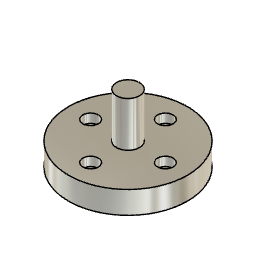
Full Assembly v48 (Autodesk Fusion 360 archive; units mm, degrees)
design "Top Cap For Metal Cylinder"
Autodesk Fusion 360 part; units mm, degrees
cylinder "CylinderPrimitive1" add diameter 50.5 height 28.575 placed x (1, 0, 0) y (0, 1, 0) z (0, 0, 1) at (0, 0, 0)
sketch "Sketch2" plane through (0, 0, 28.575) normal (0, 0, 1) x (-1, 0, 0)
  circle A0 centre (0, 0) radius 25.25
  circle A1 centre (0, 0) radius 4.9
  dimension "d3" = 9.8
  constraint concentric A0 A1
  measures "d3" diameter of A1
extrude "Extrude1" cut sketch "Sketch2" against normal blind 19.05
sketch "Sketch3" plane through (0, 0, 9.525) normal (0, 0, 1) x (-1, 0, 0)
  circle A0 centre (0, 0) radius 4.9
  circle A1 centre (0, 0) radius 25.25
  line L0 (0, 0) -> (0, 15.875)
  line L1 (0, 0) -> (15.875, 0)
  line L2 (0, 0) -> (0, -15.875)
  line L3 (0, 0) -> (-15.875, 0)
  dimension "d6" = 15.875
  dimension "d7" = 15.875
  dimension "d8" = 15.875
  dimension "d9" = 15.875
  constraint coincident A0.centre A1.centre
  constraint vertical L0
  constraint horizontal L1
  constraint vertical L2
  constraint perpendicular L2 L3
  measures "d6" distance of A0.centre L0.end
  measures "d7" distance of A0.centre L1.end
  measures "d8" distance of A0.centre L2.end
  measures "d9" distance of A0.centre L3.end
hole "Hole1" at (-15.875, 0, 9.525) at (0, 15.875, 9.525) at (0, -15.875, 9.525) at (15.875, 0, 9.525) direction (0, 0, -1) diameter 3.9 depth 16.3 tip angle 180 counterbore diameter 6.6 counterbore depth 3.8

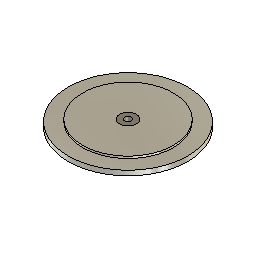
design "Top Rotary Disk"
Autodesk Fusion 360 part; units mm, degrees
sketch "Sketch1" plane through (0, 0, 0) normal (0, 0, 1) x (1, 0, 0)
  circle A0 centre (0, 0) radius 89
  circle A1 centre (0, 0) radius 67.55
  dimension "d1" = 178
  dimension "d2" = 135.1
  constraint coincident A0.centre A1.centre
  measures "d1" diameter of A0
  measures "d2" diameter of A1
extrude "Extrude1" add sketch "Sketch1" along normal blind 8 contours A1 makes body 1
extrude "Extrude2" add sketch "Sketch1" along normal blind 5 bodies 1
sketch "Sketch2" plane through (0, 0, 8) normal (0, 0, 1) x (-1, 0, 0)
  circle A0 centre (0, 0) radius 67.55
  circle A1 centre (0, 0) radius 12.5
  circle A2 centre (0, 0) radius 4.9
  dimension "d7" = 25
  dimension "d19" = 9.8
  constraint coincident A0.centre A1.centre
  measures "d7" diameter of A1
  measures "d19" diameter of A2
extrude "Extrude3" cut sketch "Sketch2" against normal blind 10 contours A1 | A2 bodies 1
sketch "Sketch3" plane through (0, 0, 0) normal (0, 0, 1) x (1, 0, 0)
  circle A0 centre (0, 0) radius 4.9
  circle A1 centre (0, 0) radius 12.5
  dimension "d10" = 9.8
  constraint coincident A0.centre A1.centre
  measures "d10" diameter of A0
extrude "Extrude5" add sketch "Sketch1" against normal blind 2.1882 contours A0 | A1 bodies 1
sketch "Sketch4" plane through (0, 0, -2.1882) normal (0, 0, -1) x (1, 0, 0)
  circle A0 centre (0, 0) radius 89
  circle A1 centre (0, 0) radius 19.05
  circle A2 centre (0, 0) radius 5.08
  dimension "d15" = 38.1
  dimension "d16" = 10.16
  constraint coincident A0.centre A1.centre
  measures "d15" diameter of A1
  measures "d16" diameter of A2
extrude "Extrude6" add sketch "Sketch4" along normal blind 12.7 contours A1 bodies 1
sketch "Sketch5" plane through (0, 0, 8) normal (0, 0, 1) x (-1, 0, 0)
  circle A0 centre (0, 0) radius 12.5
  circle A1 centre (0, 0) radius 4.9
extrude "Extrude7" add sketch "Sketch5" against normal up to surface (8 mm away) separate body makes body 2
equation "d13 = -( 0.283 in - 5 mm )"
named bodies: "Bearing"

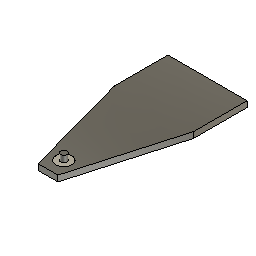
design "Top Mounting Plate"
Autodesk Fusion 360 part; units mm, degrees
sketch "Sketch1" plane through (0, 0, 0) normal (0, 0, 1) x (1, 0, 0)
  line L0 (0, 0) -> (-127, 0)
  line L1 (-127, 0) -> (-127, -85.725)
  line L2 (-127, -85.725) -> (0, -85.725)
  line L3 (0, -85.725) -> (0, 0)
  line L4 (-127, -85.725) -> (-80.1138, -255.2229)
  line L5 (0, -85.725) -> (-48.3638, -255.2229)
  line L6 (-80.1138, -255.2229) -> (-48.3638, -255.2229)
  line L7 (-64.2388, -255.2229) -> (-64.2388, -242.5229)
  line L8 (-64.2388, -242.5229) -> (-64.2388, -229.8229)
  circle A0 centre (-64.2388, -229.8229) radius 12.7
  circle A1 centre (-64.2388, -229.8229) radius 5.08
  dimension "d10" = 31.75
  dimension "d11" = 12.7
  dimension "d12" = 12.7
  dimension "d13" = 25.4
  dimension "d14" = 10.16
  dimension "d15" = 127
  dimension "d16" = 85.725
  constraint horizontal L0
  constraint vertical L1
  constraint horizontal L2
  constraint vertical L3
  constraint coincident L0.start L3.end
  constraint horizontal L6
  constraint coincident L4.end L6.start
  constraint coincident L5.end L6.end
  constraint midpoint L6 L7.start
  constraint perpendicular L6 L7
  constraint coincident L8.end A0.centre
  constraint concentric A0 A1
  measures "d10" distance of L4.end L5.end
  measures "d11" distance of L7.start L7.end
  measures "d12" distance of L7.end L8.end
  measures "d13" diameter of A0
  measures "d14" diameter of A1
  measures "d15" distance of L0.start L0.end
  measures "d16" distance of L0.start L2.end
extrude "Extrude1" add sketch "Sketch1" along normal blind 9.525 contours L0 L1 L2 L3 | L2 L4 L5 L6 makes body 1
extrude "Extrude3" add sketch "Sketch1" along normal blind 25 separate body contours A0 makes body 2
extrude "Extrude4" cut 1 faces at (-73.4515, -225.6029, 25) along direction (0, 0, -1) blind 15.475 on bodies 2 bodies 2
extrude "Extrude5" add sketch "Sketch1" along normal blind 20 separate body contours A1 makes body 3
extrude "Extrude6" add sketch "Sketch1" against normal blind 12.7 separate body contours A1 makes body 4
combine "Combine1" operation add target body 3 tool bodies 4
named bodies: "Bearing", "Axle"

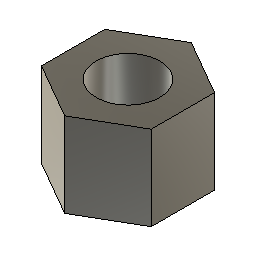
design "Hex Bolt Spacers"
Autodesk Fusion 360 part; units mm, degrees
sketch "Sketch1" plane through (0, 0, 0) normal (0, 0, 1) x (1, 0, 0)
  circle A0 centre (0, 0) radius 9.525 construction
  line L0 (0, 0) -> (0, 9.525) construction
  line L1 (0, 0) -> (8.2489, -4.7625) construction
  line L2 (0, 0) -> (-8.2489, -4.7625) construction
  line L3 (0, 0) -> (0, -9.525) construction
  line L4 (0, 0) -> (-8.2489, 4.7625) construction
  line L5 (0, 0) -> (8.2489, 4.7625) construction
  line L6 (-8.2489, 4.7625) -> (0, 9.525)
  line L7 (0, 9.525) -> (8.2489, 4.7625)
  line L8 (8.2489, 4.7625) -> (8.2489, -4.7625)
  line L9 (8.2489, -4.7625) -> (0, -9.525)
  line L10 (-8.2489, -4.7625) -> (0, -9.525)
  line L11 (-8.2489, 4.7625) -> (-8.2489, -4.7625)
  circle A1 centre (0, 0) radius 4.7625
  dimension "d1" = 19.05
  constraint coincident A0.centre L0.start
  constraint coincident A0 L0.end
  constraint vertical L0
  constraint coincident A0 L1.end
  constraint coincident A0 L3.end
  constraint vertical L3
  constraint coincident A0 L4.end
  constraint parallel L1 L4
  constraint coincident A0 L5.end
  constraint parallel L2 L5
  constraint vertical L8
  constraint parallel L7 L10
  measures "d1" diameter of A0
extrude "Extrude1" add sketch "Sketch1" along normal blind 12.7
sketch "Sketch2" plane through (0, 0, 12.7) normal (0, 0, 1) x (-1, 0, 0)
  circle A0 centre (0, 0) radius 4.7625
  line L0 (0, -9.525) -> (8.2489, -4.7625)
  line L1 (8.2489, -4.7625) -> (8.2489, 4.7625)
  line L2 (8.2489, 4.7625) -> (0, 9.525)
  line L3 (0, 9.525) -> (-8.2489, 4.7625)
  line L4 (-8.2489, 4.7625) -> (-8.2489, -4.7625)
  line L5 (-8.2489, -4.7625) -> (0, -9.525)

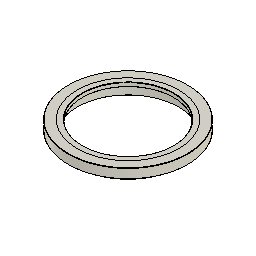
design "Top Teflon/PLA Ring"
Autodesk Fusion 360 part; units mm, degrees
sketch "Sketch1" plane through (0, 0, 0) normal (0, 0, 1) x (1, 0, 0)
  circle A0 centre (0, 0) radius 89
  dimension "d1" = 178
  constraint coincident A0.centre origin
  measures "d1" diameter of A0
extrude "Extrude1" add sketch "Sketch1" along normal blind 14.2748
sketch "Sketch2" plane through (0, 0, 0) normal (0, 0, -1) x (1, 0, 0)
  circle A0 centre (0, 0) radius 89
  circle A1 centre (0, 0) radius 78.125
  circle A2 centre (0, 0) radius 75.6231
  dimension "d4" = 156.25
  dimension "d5" = 151.2462
  constraint coincident A0.centre A1.centre
  constraint concentric A1 A2
  measures "d4" diameter of A1
  measures "d5" diameter of A2
extrude "Extrude2" add sketch "Sketch2" along normal blind 8.255 contours A1
extrude "Extrude3" cut 1 faces at (17.6402, 5.9585, 0) along direction (0, 0, 1) blind 60
sketch "Sketch3" plane through (0, 0, 0) normal (0, 0, -1) x (1, 0, 0)
  circle A0 centre (0, 0) radius 75.6231
  circle A1 centre (0, 0) radius 67.625
  dimension "d10" = 135.25
  constraint concentric A0 A1
  measures "d10" diameter of A1
extrude "Extrude4" add sketch "Sketch3" against normal blind 14.275
extrude "Extrude5" cut 1 faces at (72.4237, 7.1167, 0) along direction (0, 0, 1) blind 6
extrude "Extrude6" cut 1 faces at (72.4237, 7.1167, 6) along direction (0, 0, 1) blind 2.255
fillet "Fillet1" radius 1 1 edges at (-72.8381, -28.2512, 0)
fillet "Fillet2" radius 0.5 1 edges at (-70.5055, -27.3465, -8.255)
fillet "Fillet3" radius 0.5 1 edges at (-72.8381, 28.2512, -8.255)
fillet "Fillet4" radius 0.5 1 edges at (-70.5055, -27.3465, 8.255)
fillet "Fillet5" radius 0.5 1 edges at (-82.9771, -32.1838, 0)
fillet "Fillet6" radius 0.5 1 edges at (-82.9771, -32.1838, 14.2748)
fillet "Fillet7" radius 0.5 2 edges at (-63.0486, 24.4542, 14.275) (-63.0486, 24.4542, 8.255)
equation "d2 = 0.27 in + 0.292 in"
equation "d5 = d4 - 0.197 in"
equation "d6 = 0.625 in - 0.3 in"
equation "d15 = 6.00 mm - 0.325 in"

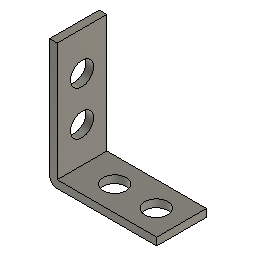
design "L bracket"
Autodesk Fusion 360 part; units mm, degrees
sketch "Sketch1" plane through (0, 0, 0) normal (0, 0, 1) x (1, 0, 0)
  line L0 (0, 0) -> (89.0778, 0)
  line L1 (89.0778, 0) -> (89.0778, 41.3004)
  line L2 (89.0778, 41.3004) -> (0, 41.3004)
  line L3 (0, 41.3004) -> (0, 0)
  line L4 (0, 41.3004) -> (6.35, 41.3004)
  line L5 (6.35, 41.3004) -> (6.35, 0)
  line L6 (6.35, 0) -> (0, 0)
  line L7 (0, 0) -> (0, 41.3004)
  circle A0 centre (33.4171, 20.6502) radius 9.525
  circle A1 centre (68.046, 20.6502) radius 9.525
  point P0 (50.7316, 20.6502)
  dimension "d1" = 89.0778
  dimension "d2" = 41.3004
  dimension "d7" = 6.35
  dimension "d12" = 19.05
  dimension "d19" = 17.3145
  dimension "d20" = 17.3145
  constraint horizontal L0
  constraint vertical L1
  constraint horizontal L2
  constraint vertical L3
  constraint coincident L0.start L3.end
  constraint horizontal L4
  constraint vertical L5
  constraint horizontal L6
  constraint vertical L7
  constraint coincident L0 L5.end
  constraint equal A0 A1
  measures "d1" distance of L0.start L0.end
  measures "d2" distance of L0.start L2.end
  measures "d7" distance of L2.end L4.end
  measures "d12" diameter of A1
  measures "d19" distance of A0.centre P0
  measures "d20" distance of A1.centre P0
extrude "Extrude1" add sketch "Sketch1" along normal blind 6.35 contours L0 L2 L3 L4 L5 L6 L7 | L0 L1 L2 L5 | A0 | A1
extrude "Extrude2" add sketch "Sketch1" along normal blind 104.648 contours L0 L2 L3 L4 L5 L6 L7
fillet "Fillet1" radius 6.35 1 edges at (0, 20.6502, 0)
extrude "Extrude3" cut sketch "Sketch1" along normal blind 129.54 contours A0 | A1
sketch "Sketch2" plane through (0, 0, 0) normal (-1, 0, 0) x (0, -1, 0)
  line L0 (-41.3004, 6.35) -> (0, 6.35)
  line L1 (0, 6.35) -> (0, 104.648)
  line L2 (0, 104.648) -> (-41.3004, 104.648)
  line L3 (-41.3004, 104.648) -> (-41.3004, 6.35)
  line L4 (-20.6502, 104.648) -> (-20.6502, 6.35) construction
  circle A0 centre (-20.6502, 72.4894) radius 9.525
  circle A1 centre (-20.6502, 35.7876) radius 9.525
  dimension "d15" = 19.05
  dimension "d16" = 19.05
  constraint midpoint L2 L4.start
  constraint midpoint L0 L4.end
  constraint coincident L4 A0.centre
  constraint coincident L4 A1.centre
  measures "d15" diameter of A0
  measures "d16" diameter of A1
extrude "Extrude4" cut sketch "Sketch2" against normal blind 182.88 contours A0 | A1
equation "d20 = d19"

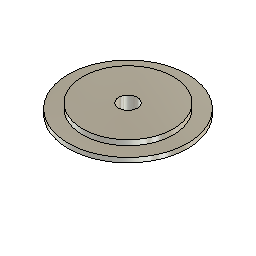
design "Bottom Rotary Disk"
Autodesk Fusion 360 part; units mm, degrees
cylinder "CylinderPrimitive1" add diameter 178 height 14.8 placed x (1, 0, 0) y (0, 1, 0) z (0, 0, 1) at (0, 0, 0) makes body 1
sketch "Sketch2" plane through (0, 0, 14.8) normal (0, 0, 1) x (-1, 0, 0)
  circle A0 centre (0, 0) radius 89
  circle A1 centre (0, 0) radius 67.55
  dimension "d3" = 135.1
  constraint concentric A0 A1
  measures "d3" diameter of A1
extrude "Extrude1" cut sketch "Sketch2" against normal blind 7.8 bodies 1
sketch "Sketch3" plane through (0, 0, 14.8) normal (0, 0, 1) x (-1, 0, 0)
  circle A0 centre (0, 0) radius 67.55
  circle A1 centre (0, 0) radius 11.75
  dimension "d6" = 23.5
  constraint coincident A0.centre A1.centre
  measures "d6" diameter of A1
sketch "Sketch4" plane through (0, 0, 0) normal (0, 0, -1) x (1, 0, 0)
  circle A0 centre (0, 0) radius 89
  circle A1 centre (0, 0) radius 24.6
  dimension "d7" = 49.2
  constraint concentric A0 A1
  measures "d7" diameter of A1
extrude "Extrude2" add sketch "Sketch4" along normal blind 11 contours A1 bodies 1
sketch "Sketch5" plane through (0, 0, -11) normal (0, 0, -1) x (1, 0, 0)
  circle A0 centre (0, 0) radius 24.6
  circle A1 centre (0, 0) radius 22.1
  dimension "d10" = 44.2
  constraint coincident A0.centre A1.centre
  measures "d10" diameter of A1
extrude "Extrude3" add sketch "Sketch5" along normal blind 27.5 contours A1 bodies 1
sketch "Sketch6" plane through (0, 0, -38.5) normal (0, 0, -1) x (1, 0, 0)
  circle A0 centre (0, 0) radius 22.1
  circle A1 centre (0, 0) radius 12.65
  dimension "d13" = 25.3
  constraint coincident A0.centre A1.centre
  measures "d13" diameter of A1
extrude "Extrude4" add sketch "Sketch6" along normal blind 12 contours A1 bodies 1
sketch "Sketch9" plane through (0, 0, 0) normal (0, 0, 1) x (1, 0, 0)
  line L0 (100, 160) -> (100, 164.1)
  line L1 (100, 176) -> (100, 171.9)
  line L2 (101.85, 176) -> (100, 176)
  line L3 (101.85, 160) -> (100, 160)
  arc A0 (100, 164.1) -> (100, 171.9) centre (96.8142, 168) ccw
  line L4 (100, 160) -> (105.45, 160)
  line L5 (105.45, 176) -> (101.85, 176)
  line L6 (100, 176) -> (125.6, 176)
  line L7 (125.6, 176) -> (125.6, 160)
  line L8 (125.6, 160) -> (105.45, 160)
  dimension "d16" = 4.1
  dimension "d17" = 16
  dimension "d19" = 4.1
  dimension "d21" = 25.6
  constraint vertical L0
  constraint vertical L1
  constraint horizontal L4
  constraint horizontal L6
  constraint perpendicular L6 L7
  measures "d16" distance of L0.start L0.end
  measures "d17" distance of L0.start L1.start
  measures "d19" distance of L1.start L1.end
  measures "d21" distance of L1.start L6.end
sketch "Sketch10" plane through (0, 176, 0) normal (0, 1, 0) x (-1, 0, 0)
  circle A0 centre (-125.6, 0) radius 25.6
  circle A1 centre (-125.6, 0) radius 22.2
  dimension "d23" = 44.4
  constraint concentric A0 A1
  measures "d23" diameter of A1
copy_body "Body->Comp2" bodies 1 removing the originals makes body 2 in component "plate"
sketch "Sketch11" plane through (0, 0, 14.8) normal (0, 0, 1) x (-1, 0, 0)
  circle A0 centre (0, 0) radius 67.55
  circle A1 centre (0, 0) radius 13.95
  circle A2 centre (0, 0) radius 6
  dimension "d34" = 27.9
  dimension "d35" = 12
  constraint concentric A0 A1
  constraint concentric A1 A2
  measures "d34" diameter of A1
  measures "d35" diameter of A2
extrude "Extrude1'" cut sketch "Sketch11" against normal blind 185 contours A2 bodies 2 in component "plate"
extrude "Extrude2'" cut sketch "Sketch11" against normal blind 25 contours A1 bodies 2 in component "plate"
component "plate" placed x (1, 0, 0) y (0, 1, 0) z (0, 0, 1) at (0, 0, 0)
equation "d21 = ( 51.2 / 2 ) * 1 mm"

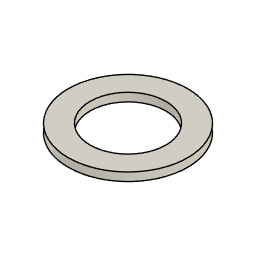
design "Spacing Washer"
Autodesk Fusion 360 part; units mm, degrees
sketch "Sketch1" plane through (0, 0, 0) normal (0, 0, 1) x (1, 0, 0)
  circle A0 centre (0, 0) radius 23.1775
  circle A1 centre (0, 0) radius 36.576
  dimension "d1" = 46.355
  dimension "d2" = 73.152
  constraint coincident A0.centre A1.centre
  measures "d1" diameter of A0
  measures "d2" diameter of A1
extrude "Extrude1" add sketch "Sketch1" along normal blind 5.08
equation "d3 = 2.54 * 2 mm"

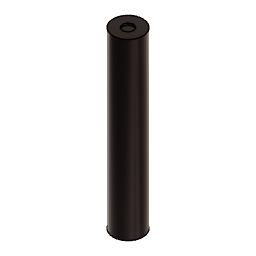
design "Inner Metal Cylinder"
Autodesk Fusion 360 part; units mm, degrees
sketch "Sketch2" plane through (0, 0, 0) normal (0, 0, 1) x (1, 0, 0)
cylinder "CylinderPrimitive2" add diameter 137.3 height 804.8625 placed x (1, 0, 0) y (0, 1, 0) z (0, 0, 1) at (0, 0, 0)
sketch "Sketch3" plane through (0, 0, 804.8625) normal (0, 0, 1) x (-1, 0, 0)
  circle A0 centre (0, 0) radius 68.65
  circle A1 centre (0, 0) radius 25.25
  dimension "d5" = 50.5
  constraint coincident A0.centre A1.centre
  measures "d5" diameter of A1
extrude "Extrude1" cut sketch "Sketch3" against normal blind 28.575 contours A1
sketch "Sketch4" plane through (0, 0, 0) normal (0, 0, 1) x (1, 0, 0)
  circle A0 centre (0, 0) radius 25.25
  dimension "d8" = 50.5
  constraint coincident A0.centre origin
  measures "d8" diameter of A0
extrude "Extrude2" cut sketch "Sketch4" along normal blind 28.575
extrude "Extrude3" add 1 faces at (-8.0427, -2.4809, 776.2875) along direction (0, 0, 1) blind 28.575
extrude "Extrude4" add 1 faces at (4.2083, -8.3807, 28.575) along direction (0, 0, -1) blind 28.575
extrude "Extrude5" cut sketch "Sketch3" against normal blind 9.25 contours A1
extrude "Extrude6" cut sketch "Sketch4" along normal blind 9.25
equation "d3 = 31 11/16\""

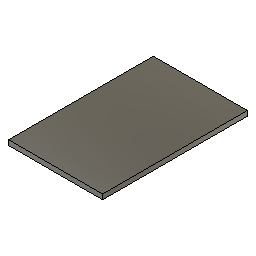
design "Bottom Standing Plate"
Autodesk Fusion 360 part; units mm, degrees
sketch "Sketch1" plane through (0, 0, 0) normal (0, 0, 1) x (1, 0, 0)
  line L0 (0, 0) -> (358.775, 0)
  line L1 (358.775, 0) -> (358.775, -552.45)
  line L2 (358.775, -552.45) -> (0, -552.45)
  line L3 (0, -552.45) -> (0, 0)
  dimension "d3" = 552.45
  dimension "d4" = 358.775
  constraint horizontal L0
  constraint vertical L1
  constraint horizontal L2
  constraint vertical L3
  constraint coincident L0.start L3.end
  measures "d3" distance of L0.start L2.end
  measures "d4" distance of L0.start L0.end
extrude "Extrude1" add sketch "Sketch1" along normal blind 19.05

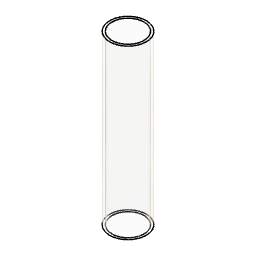
design "Clear Acrylic Tube"
Autodesk Fusion 360 part; units mm, degrees
cylinder "CylinderPrimitive1" add diameter 177.8 height 814.3875 placed x (1, 0, 0) y (0, 1, 0) z (0, 0, 1) at (0, 0, 0)
sketch "Sketch2" plane through (0, 0, 0) normal (0, 0, 1) x (1, 0, 0)
  circle A0 centre (0, 0) radius 77.7875
  dimension "d3" = 155.575
  constraint coincident A0.centre origin
  measures "d3" diameter of A0
extrude "Extrude1" cut sketch "Sketch2" along normal blind 1016
equation "d1 = 32 1/16\""

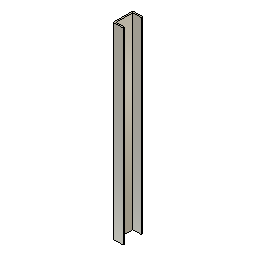
design "Steel Standing Bracket"
Autodesk Fusion 360 part; units mm, degrees
sketch "Sketch1" plane through (0, 0, 0) normal (0, 0, 1) x (1, 0, 0)
  line L0 (0, 0) -> (21.0566, 0)
  line L1 (21.0566, 0) -> (21.0566, 41.3258)
  line L2 (21.0566, 41.3258) -> (0, 41.3258)
  line L3 (0, 41.3258) -> (0, 0)
  line L4 (0, 20.6629) -> (21.0566, 20.6629) construction
  line L5 (0, 38.1508) -> (21.0566, 38.1508)
  line L6 (21.0566, 38.1508) -> (21.0566, 3.175) construction
  line L7 (21.0566, 3.175) -> (0, 3.175)
  line L8 (0, 3.175) -> (0, 38.1508) construction
  line L9 (0, 38.1508) -> (21.0566, 3.175) construction
  line L10 (21.0566, 38.1508) -> (0, 3.175) construction
  line L11 (3.175, 38.1508) -> (3.175, 3.175)
  point P0 (10.5283, 20.6629)
  point P1 (0, 20.6629)
  dimension "d1" = 41.3258
  dimension "d2" = 21.0566
  dimension "d3" = 3.175
  dimension "d4" = 3.175
  constraint horizontal L0
  constraint vertical L1
  constraint horizontal L2
  constraint vertical L3
  constraint coincident L0.start L3.end
  constraint midpoint L3 P1
  constraint midpoint L1 L4.end
  constraint horizontal L5
  constraint perpendicular L5 L6
  constraint parallel L5 L7
  constraint parallel L6 L8
  constraint coincident L9 P0
  constraint coincident L10 P0
  constraint coincident L3 L5.start
  constraint midpoint L4 P0
  constraint coincident L5 L11.start
  constraint coincident L7 L11.end
  constraint perpendicular L7 L11
  constraint coincident P1 L4.start
  measures "d1" distance of L0.start L2.end
  measures "d2" distance of L1.end L2.end
  measures "d3" distance of L3 L11
  measures "d4" distance of L2 L5
extrude "Extrude1" add sketch "Sketch1" along normal blind 395 contours L0 L1 L3 L7 | L3 L5 L7 L11 | L1 L2 L3 L5
sketch "Sketch2" plane through (0, 0, 395) normal (0, 0, 1) x (-1, 0, 0)
  line L0 (-21.0566, -38.1508) -> (-21.0566, -41.3258)
  line L1 (-21.0566, -41.3258) -> (0, -41.3258)
  line L2 (0, -41.3258) -> (0, 0)
  line L3 (0, 0) -> (-21.0566, 0)
  line L4 (-21.0566, 0) -> (-21.0566, -3.175)
  line L5 (-21.0566, -3.175) -> (-3.175, -3.175)
  line L6 (-3.175, -3.175) -> (-3.175, -38.1508)
  line L7 (-3.175, -38.1508) -> (-21.0566, -38.1508)
  point P0 (0, -20.6629)

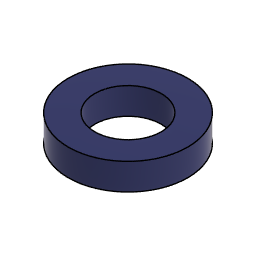
design "Small Seal"
Autodesk Fusion 360 part; units mm, degrees
sketch "Sketch1" plane through (0, 0, 0) normal (0, 0, 1) x (1, 0, 0)
  circle A0 centre (0, 0) radius 7.94
  circle A1 centre (0, 0) radius 14.275
  dimension "d1" = 15.88
  dimension "d2" = 28.55
  constraint coincident A0.centre A1.centre
  constraint concentric A0 A1
  measures "d1" diameter of A0
  measures "d2" diameter of A1
extrude "Extrude1" add sketch "Sketch1" along normal blind 6.35

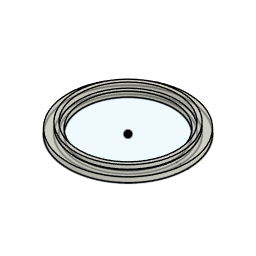
design "Bottom Teflon Ring"
Autodesk Fusion 360 part; units mm, degrees
sketch "Sketch1" plane through (0, 0, 0) normal (0, 0, 1) x (1, 0, 0)
  circle A0 centre (0, 0) radius 67.4
  circle A1 centre (0, 0) radius 89
  circle A2 centre (0, 0) radius 72.8
  circle A3 centre (0, 0) radius 78.05
  dimension "d1" = 134.8
  dimension "d2" = 178
  dimension "d3" = 145.6
  dimension "d4" = 156.1
  constraint coincident A0.centre A1.centre
  constraint concentric A0 A1
  measures "d1" diameter of A0
  measures "d2" diameter of A1
  measures "d3" diameter of A2
  measures "d4" diameter of A3
extrude "Extrude1" add sketch "Sketch1" along normal blind 7.7 contours A1 makes body 1
extrude "Extrude2" add sketch "Sketch1" along normal blind 7.7 separate body contours A2 makes body 2
extrude "Extrude4" add sketch "Sketch1" along normal blind 15.6 contours A3 bodies 1 2
sketch "Sketch3" plane through (0, 0, 7.7) normal (0, 0, 1) x (-1, 0, 0)
  circle A0 centre (0, 0) radius 78.05
  circle A1 centre (0, 0) radius 89
  circle A2 centre (0, 0) radius 76.55
  circle A3 centre (0, 0) radius 77.8
  dimension "d13" = 153.1
  constraint coincident A0.centre A1.centre
  constraint concentric A2 A3
  measures "d13" diameter of A2
extrude "Extrude5" cut sketch "Sketch3" along normal blind 2 contours A0 | A3 bodies 1
extrude "Extrude3" [suppressed]
equation "d2 = 135 mm + ( 21.8 * 2 ) * 1 mm - 0.6 mm"
equation "d4 = 145.600 mm + 10.5 mm"
equation "d13 = 155.600 mm - 2.5 mm"

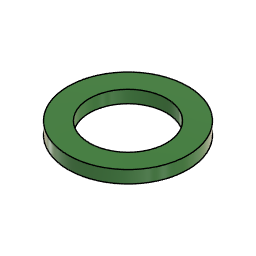
design "Big Seal"
Autodesk Fusion 360 part; units mm, degrees
sketch "Sketch1" plane through (0, 0, 0) normal (0, 0, 1) x (1, 0, 0)
  circle A0 centre (0, 0) radius 24.615
  circle A1 centre (0, 0) radius 38.1
  dimension "d1" = 49.23
  dimension "d2" = 76.2
  constraint coincident A0.centre A1.centre
  measures "d1" diameter of A0
  measures "d2" diameter of A1
extrude "Extrude1" add sketch "Sketch1" along normal blind 7.95
